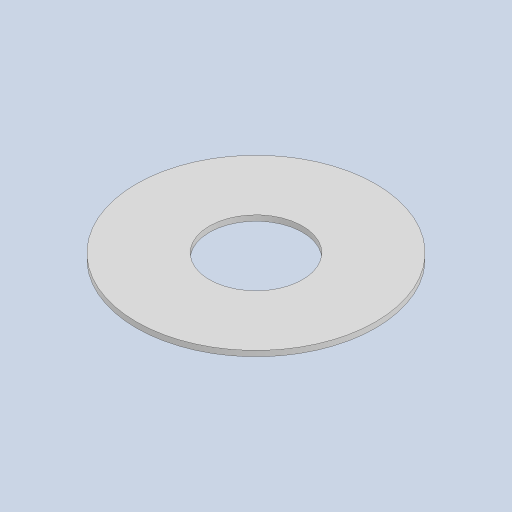
# Autodesk Inventor part: upper card holder
Saved by Autodesk Inventor 2023 (Build 270158000, 158)
## iProperties
Created: 2023-06-01
Part Number: upper card holder
Material: Generic
Document SubType Name: Modeling
Designer: cheng
Density: 1 g/cm^3
Appearance: Default
Author: cheng
Autodesk Inventor part; units mm, degrees
ref_plane "YZ Plane" through (0, 0, 0) normal (1, 0, 0) x (0, 1, 0)
ref_plane "XZ Plane" through (0, 0, 0) normal (0, 1, 0) x (-1, 0, 0)
ref_plane "XY Plane" through (0, 0, 0) normal (0, 0, 1) x (1, 0, 0)
sketch "Sketch1" plane through (0, 0, 0) normal (0, 1, 0) x (-1, 0, 0)
  circle A0 centre (0, 0) radius 65.5
  circle A1 centre (0, 0) radius 25.5
  dimension "d0" = 51
  dimension "d1" = 40
  constraints: 2 centre point, 2 coincident
  measures "d0" diameter of A1
  measures "d1" radial gap between concentric circles of A0 A1
extrude "Extrusion1" add sketch "Sketch1" along normal blind 3
body "Solid1"
